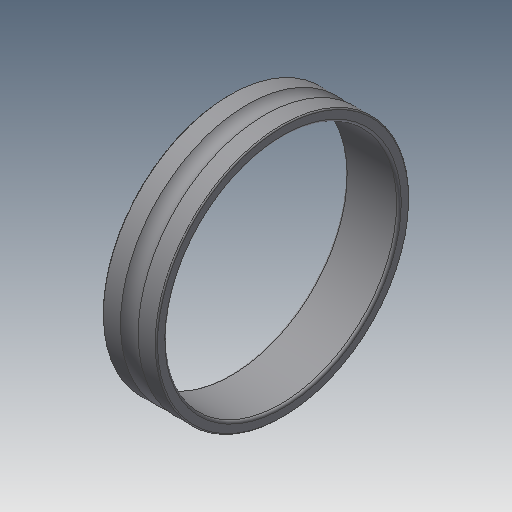
# Autodesk Inventor part: A-2015_ir
Saved by Autodesk Inventor 2019.4 (Build 234330000, 330)
## iProperties
Category: PARTsolutions
Company: NMB
Created: 2019-11-12
Part Number: A-2015_ir
Material: 一般
Catalog Web Link: www.cadenas.de
Description: Radial Ball Bearings (A series)  OT ir-Radial Ball Bearings (A series)  Open Type
Vendor: NMB
Document SubType Name: Modeling
Designer: psadmin
Manufacturer: NMB
Mass: 0.110457 g
Surface Area: 4.10544 cm^2
Volume: 0.110457 cm^3
Density: 1 g/cm^3
Appearance: PSOLRGB-192-192-192
PSOL_IDENT_0: {$CADENAS_DATA\23d-libs\nmb\pbbp\radial_ball_bear_thin_secti\rbb_as\as_open_ir.prj},191 {VTYP=3D},{N
PSOL_IDENT_1: B=A-2015_ir},{LINA=A-2015_ir},{NN=Radial Ball Bearings (A series)  OT ir},{DATE=11.11.2013 05:13:38}
PSOL_IDENT_2: ,{GEOMDATE=29.10.2013 14:08:00},{VERSION=},{LINEID=870},{WBVAR=},{WBNUMERIC=}  {NB=A-2015_ir},{LINA=
PSOL_IDENT_3: A-2015_ir},{KT=DUMMY},{IDNR=},{PN=A-2015},{SHLD=open},{FLANG=unflanged},{SD=15.000},{D=20.000},{B=3.
PSOL_IDENT_4: 500},{SR=0.15},{BCZ=14},{DW=1.5875},{LI=16.40},{LO=18.43},{D1=0.000},{C1=0.00},{D2=0.0},{C2=0.00},{C
PSOL_IDENT_5: OR=582},{CR=1085},{PCD=17.500},{U=19.088},{W=15.913},{Y=0.794},{Z=0.794},{AA=0.000},{AC=0.00},{AD=0.
PSOL_IDENT_6: 000},{AF=0.00},{AQ=0.00},{AH=0.00},{AI=0.00},{AJ=0.00}
NN: Radial Ball Bearings (A series)  OT ir
NT: Radial Ball Bearings (A series)  Open Type
NB: A-2015_ir
NBSYN: $PN._ir
LINA: A-2015_ir
PN: A-2015
SHLD: open
FLANG: unflanged
SD: 15
D: 20
B: 3.5
SR: 0.15
BCZ: 14
DW: 1.5875
LI: 16.4
LO: 18.43
D1: 0
C1: 0
D2: 0
C2: 0
COR: 582
CR: 1085
PCD: 17.5
U: 19.088
W: 15.913
Y: 0.794
Z: 0.794
AA: 0
AC: 0
AD: 0
AF: 0
AQ: 0
AH: 0
AI: 0
AJ: 0
SUPPLIER: NMB
ARTICLENO: A-2015_ir
BOMINFO: A-2015_ir
CREATOR: CADENAS GmbH
Title: A-2015_ir
Author: Cadenas PARTsolutions
Comments: Radial Ball Bearings (A series)  Open Type
Autodesk Inventor part; units mm, degrees
sketch "Sketch_1" plane through (0, 0, 0) normal (0, 0, 1) x (1, 0, 0)
  line L0 (3.5, 0) -> (0, 0)
  line L1 (0, 8.125) -> (0, 7.65)
  arc A0 (0, 7.65) -> (0.15, 7.5) centre (0.15, 7.65) ccw
  line L2 (0.15, 7.5) -> (3.35, 7.5)
  arc A1 (3.35, 7.5) -> (3.5, 7.65) centre (3.35, 7.65) ccw
  line L3 (3.5, 7.65) -> (3.5, 8.125)
  arc A2 (3.5, 8.125) -> (3.425, 8.2) centre (3.425, 8.125) ccw
  line L4 (3.425, 8.2) -> (2.3223, 8.2)
  arc A3 (1.1777, 8.2) -> (2.3223, 8.2) centre (1.75, 8.75) ccw
  line L5 (1.1777, 8.2) -> (0.075, 8.2)
  arc A4 (0.075, 8.2) -> (0, 8.125) centre (0.075, 8.125) ccw
  constraints: 12 end point, 10 point on circle, 5 centre point
revolve "Revolution1" add sketch "Sketch_1" angle 360 about axis through (3.5, 0, 0) along (1, 0, 0)
ref_plane "1_XY" through (1.75, 0, 0) normal (1, 0, 0) x (0, 0, -1)
ref_plane "1_YZ" through (1.75, 0, 0) normal (0, 0, -1) x (0, 1, 0)
ref_plane "1_ZX" through (1.75, 0, 0) normal (0, 1, 0) x (1, 0, 0)
ref_plane "1_Dummy_XY" through (0, 0, 0) normal (-1, 0, 0) x (0, 0, -1)
ref_plane "1_Dummy_YZ" through (0, 0, 0) normal (0, 0, -1) x (0, -1, 0)
ref_plane "1_Dummy_ZX" through (0, 0, 0) normal (0, -1, 0) x (-1, 0, 0)
body "Solid1"
